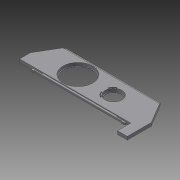
# Autodesk Inventor part: Ti Transmitted Slider
Saved by Autodesk Inventor 2013 (Build 170138000, 138)
## iProperties
Created: 2013-06-03
Part Number: Ti Transmitted Slider
Material: Generic
Document SubType Name: Modeling
Designer: kthorn
Density: 1 g/cm^3
Author: kthorn
Autodesk Inventor part; units mm, degrees
ref_plane "YZ Plane" through (0, 0, 0) normal (1, 0, 0) x (0, 1, 0)
ref_plane "XZ Plane" through (0, 0, 0) normal (0, 1, 0) x (-1, 0, 0)
ref_plane "XY Plane" through (0, 0, 0) normal (0, 0, 1) x (1, 0, 0)
sketch "Sketch1" plane through (0, 0, 0) normal (0, 0, 1) x (1, 0, 0)
  line L0 (165.1282, -41.3427) -> (-17.8718, -41.3427)
  line L1 (-17.8718, -41.3427) -> (-17.8718, -25.1427)
  line L2 (2.1282, 8.6573) -> (145.1282, 8.6573)
  line L3 (165.1282, -25.1427) -> (165.1282, -41.3427)
  line L4 (-17.8718, -25.1427) -> (2.1282, 8.6573)
  line L5 (73.6282, -41.3427) -> (73.6282, 8.6573) construction
  line L6 (165.1282, -25.1427) -> (145.1282, 8.6573)
  line L7 (165.1282, -41.3427) -> (150.3282, -41.3427)
  line L8 (150.3282, -41.3427) -> (150.3282, -61.3427)
  line L9 (150.3282, -61.3427) -> (165.1282, -61.3427)
  line L10 (165.1282, -61.3427) -> (165.1282, -41.3427)
  point P0 (0, 0)
  dimension "d2" = 16.2
  dimension "d4" = 143
  dimension "d5" = 183
  dimension "d6" = 50
  dimension "d7" = 14.8
  dimension "d8" = 20
  constraints: 22 end point, 4 parallel, 2 horizontal, 2 midpoint, 2 perpendicular, 2 symmetric about line
  measures "d2" distance of L1.end L0.end
  measures "d4" distance of L2.start L2.end
  measures "d5" distance of L0.start L0.end
  measures "d6" distance between parallel lines of L0 L2
  measures "d7" distance of L8.end L9.end
  measures "d8" distance of L7.end L8.end
extrude "Extrusion1" add sketch "Sketch1" along normal blind 5
sketch "Sketch2" plane through (0, 0, 5) normal (0, 0, 1) x (1, 0, 0)
  line L0 (165.1282, -25.1427) -> (145.1282, 8.6573) projected
  line L1 (145.1282, 8.6573) -> (2.1282, 8.6573) projected
  line L2 (2.1282, 8.6573) -> (-17.8718, -25.1427) projected
  line L3 (2.1282, 8.6573) -> (145.1282, 8.6573)
  line L4 (146.7554, 5.9073) -> (0.5009, 5.9073)
  line L5 (2.1282, 8.6573) -> (0.5009, 5.9073)
  line L6 (145.1282, 8.6573) -> (146.7554, 5.9073)
  point P0 (0, 0)
  dimension "d11" = 2.75
  constraints: 8 end point, 3 point on line, 2 collinear, 1 horizontal, 1 parallel
  measures "d11" distance between parallel lines of L4 L1
extrude "Extrusion2" cut sketch "Sketch2" against normal blind 1.2
sketch "Sketch3" plane through (0, 0, 0) normal (0, 0, -1) x (-1, 0, 0)
  line L0 (-2.1282, 8.6573) -> (17.8718, -25.1427) projected
  line L1 (-145.1282, 8.6573) -> (-2.1282, 8.6573) projected
  line L2 (-165.1282, -25.1427) -> (-145.1282, 8.6573) projected
  line L3 (-145.1282, 8.6573) -> (-2.1282, 8.6573)
  line L4 (-0.5009, 5.9073) -> (-146.7554, 5.9073)
  dimension "d17" = 2.75
  constraints: 4 end point, 2 point on line, 1 collinear, 1 parallel
  measures "d17" distance between parallel lines of L3 L4
extrude "Extrusion3" cut sketch "Sketch3" against normal blind 1.2
sketch "Sketch4" plane through (-17.8718, -41.3427, 0) normal (0, -1, 0) x (1, 0, 0)
  line L0 (163, 3.8) -> (20, 3.8)
  line L1 (20, 3.8) -> (20, 1.2)
  line L2 (20, 1.2) -> (163, 1.2)
  line L3 (163, 1.2) -> (163, 3.8)
  line L4 (163, 3.8) -> (20, 1.2) construction
  line L5 (20, 3.8) -> (163, 1.2) construction
  line L6 (168.2, 0) -> (183, 0) projected
  line L7 (183, 0) -> (183, 5) projected
  line L8 (168.2, 5) -> (183, 5) projected
  line L9 (168.2, 0) -> (168.2, 5) projected
  line L10 (168.2, 5) -> (183, 5) projected
  line L11 (0, 0) -> (183, 5) construction
  line L12 (183, 0) -> (0, 5) construction
  point P0 (17.8718, 0)
  point P1 (91.5, 2.5)
  point P2 (91.5, 2.5)
  dimension "d20" = 2.6
  dimension "d22" = 143
  constraints: 16 end point, 4 midpoint, 2 parallel, 1 horizontal, 1 perpendicular
  measures "d20" distance of L0.end L1.end
  measures "d22" distance of L0.start L0.end
extrude "Extrusion4" add sketch "Sketch4" along normal blind 3.8 contours L3 L2 L1 L0
sketch "Sketch5" plane through (2.1282, -41.3427, 3.8) normal (0, 0, 1) x (1, 0, 0)
  line L0 (0, 0) -> (143, 0) projected
  line L1 (0, 0) -> (0, -3.8) projected
  line L2 (143, -3.8) -> (0, -3.8) projected
  line L3 (143, 0) -> (143, -3.8) projected
  line L4 (5.125, -3.8) -> (137.875, -3.8)
  line L5 (137.875, -3.8) -> (137.875, -2.8)
  line L6 (137.875, -2.8) -> (5.125, -2.8)
  line L7 (5.125, -2.8) -> (5.125, -3.8)
  line L8 (5.125, -2.8) -> (0, -2.8) construction
  line L9 (137.875, -2.8) -> (143, -2.8) construction
  line L10 (143, 0) -> (128, 0)
  line L11 (128, 0) -> (128, -1.25)
  line L12 (128, -1.25) -> (143, -1.25)
  line L13 (143, -1.25) -> (143, 0)
  line L14 (71.5, 0) -> (71.5, -28.6928) construction
  line L15 (0, 0) -> (15, 0)
  line L16 (15, 0) -> (15, -1.25)
  line L17 (15, -1.25) -> (0, -1.25)
  line L18 (0, -1.25) -> (0, 0)
  line L19 (143, -2.4854) -> (140.4375, -3.8)
  line L20 (140.4375, -3.8) -> (143, -3.8)
  line L21 (143, -2.4854) -> (143, -3.8)
  line L22 (0, -2.4854) -> (2.5625, -3.8)
  line L23 (2.5625, -3.8) -> (0, -3.8)
  line L24 (0, -2.4854) -> (0, -3.8)
  point P0 (-2.1282, 41.3427)
  dimension "d25" = 1
  dimension "d27" = 132.75
  dimension "d28" = 15
  dimension "d29" = 1.25
  constraints: 42 end point, 5 parallel, 5 perpendicular, 5 point on line, 5 symmetric about line, 2 collinear, 2 horizontal, 1 midpoint
  measures "d25" distance of L6.end L4.start
  measures "d27" distance of L5.end L6.end
  measures "d28" distance of L0.end L10.end
  measures "d29" distance of L10.end L11.end
extrude "Extrusion5" cut sketch "Sketch5" against normal through all contours L0 L16 L17 L1 | L0 L3 L12 L11 | L22 L2 L1 | L7 L6 L5 L2 | L3 L2 L19
sketch "Sketch6" plane through (0, 0, 5) normal (0, 0, 1) x (1, 0, 0)
  line L0 (-17.8718, -25.1427) -> (-17.8718, -41.3427) projected
  line L1 (165.1282, -61.3427) -> (165.1282, -25.1427) projected
  line L2 (-17.8718, -41.3427) -> (165.1282, -41.3427) construction
  line L3 (165.1282, -41.3427) -> (165.1282, 5.9073) construction
  line L4 (165.1282, 5.9073) -> (-17.8718, 5.9073) construction
  line L5 (-17.8718, 5.9073) -> (-17.8718, -41.3427) construction
  line L6 (-17.8718, 5.9073) -> (165.1282, -41.3427) construction
  line L7 (-17.8718, -41.3427) -> (165.1282, 5.9073) construction
  circle A0 centre (46.6282, -17.7177) radius 22.5
  circle A1 centre (100.6282, -17.7177) radius 12.75
  line L8 (-17.8718, -17.7177) -> (165.1282, -17.7177) construction
  line L9 (46.6282, -17.7177) -> (46.6282, -36.6137) construction
  line L10 (46.6282, -36.6137) -> (-17.8718, -36.6137) construction
  line L11 (100.6282, -17.7177) -> (100.6282, -34.8345) construction
  line L12 (100.6282, -34.8345) -> (165.1282, -34.8345) construction
  circle A2 centre (46.6282, -17.7177) radius 21.5
  circle A3 centre (100.6282, -17.7177) radius 11.75
  line L13 (46.6282, 3.7823) -> (46.6282, 4.7823) construction
  line L14 (100.6282, -5.9677) -> (100.6282, -4.9677) construction
  point P0 (0, 0)
  point P1 (73.6282, -17.7177)
  dimension "d32" = 45
  dimension "d35" = 25.5
  dimension "d37" = 64.5
  dimension "d38" = 64.5
  dimension "d39" = 1
  dimension "d40" = 1
  dimension "d87" = 27
  constraints: 26 end point, 6 perpendicular, 4 point on line, 4 vertical alignment, 3 midpoint, 3 parallel, 2 coincident, 1 horizontal, 8 other
  measures "d37" distance of L9.end L10.end
  measures "d38" distance of L11.end L12.end
  measures "d39" distance of L13.start L13.end
  measures "d40" distance of L14.start L14.end
  measures "d87" distance of point (73.628, -17.718) L9.start
extrude "Extrusion6" cut sketch "Sketch6" against normal through all contours A2 | A3
extrude "Extrusion7" cut sketch "Sketch6" against normal blind 4.5
sketch "Sketch11" plane through (0, 0, 5) normal (0, 0, 1) x (1, 0, 0)
  circle A0 centre (100.6282, -17.7177) radius 12.75 projected
  line L0 (165.1282, -61.3427) -> (165.1282, -25.1427) projected
  circle A1 centre (100.6282, -17.7177) radius 13.75 construction
  circle A2 centre (100.6282, -17.7177) radius 14.75 construction
  line L1 (100.6282, -17.7177) -> (93.2532, -4.9439) construction
  line L2 (100.6282, -17.7177) -> (142.9654, -17.7177) construction
  line L3 (100.6282, -17.7177) -> (93.2532, -30.4916) construction
  line L4 (100.6282, -17.7177) -> (86.7677, -22.7625) construction
  line L5 (100.6282, -17.7177) -> (86.7677, -12.673) construction
  line L6 (93.7532, -5.8099) -> (93.2532, -4.9439)
  line L7 (87.7074, -13.015) -> (86.7677, -12.673)
  line L8 (87.7074, -22.4205) -> (86.7677, -22.7625)
  line L9 (93.7532, -29.6256) -> (93.2532, -30.4916)
  arc A3 (86.7677, -22.7625) -> (93.2532, -30.4916) centre (100.6282, -17.7177) ccw
  arc A4 (87.7074, -22.4205) -> (93.7532, -29.6256) centre (100.6282, -17.7177) ccw
  arc A5 (93.7532, -5.8099) -> (87.7074, -13.015) centre (100.6282, -17.7177) ccw
  arc A6 (93.2532, -4.9439) -> (86.7677, -12.673) centre (100.6282, -17.7177) ccw
  point P0 (0, 0)
  dimension "d88" = 1
  dimension "d89" = 1
  dimension "d90" = 120
  dimension "d93" = 120
  dimension "d94" = 40
  dimension "d95" = 40
  constraints: 18 end point, 16 point on circle, 6 centre point, 6 coincident, 4 collinear, 4 point on line, 1 perpendicular
  measures "d88" radial gap between concentric circles of A0 A1
  measures "d89" radial gap between concentric circles of A2 A1
  measures "d90" angle of L1 L2
  measures "d93" angle of L3 L2
  measures "d94" angle of L1 L5
  measures "d95" angle of L3 L4
extrude "Extrusion13" cut sketch "Sketch11" against normal through all contours A5 L7 A6 L6 | A4 L9 A3 L8
sketch "Sketch12" plane through (0, 0, 5) normal (0, 0, 1) x (1, 0, 0)
  arc A0 (93.2532, -4.9439) -> (86.7677, -12.673) centre (100.6282, -17.7177) ccw projected
  line L0 (93.2532, -4.9439) -> (93.7532, -5.8099) projected
  line L1 (93.7532, -29.6256) -> (93.2532, -30.4916) projected
  arc A1 (86.7677, -22.7625) -> (93.2532, -30.4916) centre (100.6282, -17.7177) ccw projected
  circle A2 centre (100.6282, -17.7177) radius 12.75 projected
  line L2 (100.6282, -17.7177) -> (93.2532, -4.9439) construction
  line L3 (100.6282, -17.7177) -> (93.2532, -30.4916) construction
  line L4 (100.6282, -17.7177) -> (92.3801, -5.4894) construction
  line L5 (100.6282, -17.7177) -> (92.3801, -29.9461) construction
  circle A3 centre (100.6282, -17.7177) radius 11.75 construction
  line L6 (92.3801, -5.4894) -> (94.0577, -7.9766)
  line L7 (94.7532, -7.542) -> (93.2532, -4.9439)
  line L8 (93.2532, -30.4916) -> (94.7532, -27.8935)
  line L9 (92.3801, -29.9461) -> (94.0577, -27.4589)
  arc A4 (94.0577, -27.4589) -> (94.7532, -27.8935) centre (100.6282, -17.7177) ccw
  arc A5 (92.3801, -29.9461) -> (93.2532, -30.4916) centre (100.6282, -17.7177) ccw
  arc A6 (94.7532, -7.542) -> (94.0577, -7.9766) centre (100.6282, -17.7177) ccw
  arc A7 (93.2532, -4.9439) -> (92.3801, -5.4894) centre (100.6282, -17.7177) ccw
  point P0 (0, 0)
  dimension "d100" = 4
  dimension "d101" = 4
  constraints: 16 end point, 14 point on circle, 4 centre point, 4 coincident, 4 point on line, 3 collinear
  measures "d100" angle of L2 L4
  measures "d101" angle of L5 L3
extrude "Extrusion14" cut sketch "Sketch12" against normal through all contours L0 L7 A2 L6 A0 | A2 L7 A6 L6 | L9 A4 L8 A2 | A2 L8 L1 A1 L9
sketch "Sketch13" plane through (0, 0, 5) normal (0, 0, 1) x (1, 0, 0)
  arc A0 (92.9393, -6.3185) -> (87.7074, -13.015) centre (100.6282, -17.7177) ccw projected
  arc A1 (94.2532, -28.7596) -> (94.2532, -6.6759) centre (100.6282, -17.7177) ccw projected
  line L0 (100.6282, -17.7177) -> (92.9393, -6.3185) construction
  line L1 (100.6282, -17.7177) -> (91.7898, -7.1846) construction
  line L2 (100.6282, -17.7177) -> (92.9393, -29.117) construction
  line L3 (100.6282, -17.7177) -> (91.7898, -28.2509) construction
  line L4 (100.6282, -17.7177) -> (113.3782, -17.7177) construction
  line L5 (100.6282, -17.7177) -> (113.3607, -17.0505) construction
  line L6 (100.6282, -17.7177) -> (113.3607, -18.385) construction
  line L7 (113.3607, -18.385) -> (112.3621, -18.3327)
  line L8 (113.3607, -17.0505) -> (112.3621, -17.1028)
  line L9 (93.4985, -28.288) -> (94.0577, -27.4589) construction
  arc A2 (94.0577, -7.9766) -> (94.0577, -27.4589) centre (100.6282, -17.7177) ccw construction
  line L10 (94.0577, -7.9766) -> (93.4985, -7.1475) construction
  arc A3 (93.4985, -7.1475) -> (93.4985, -28.288) centre (100.6282, -17.7177) ccw construction
  line L11 (94.7532, -27.8935) -> (94.2532, -28.7596) construction
  arc A4 (94.2532, -28.7596) -> (94.2532, -6.6759) centre (100.6282, -17.7177) ccw construction
  line L12 (94.2532, -6.6759) -> (94.7532, -7.542) construction
  arc A5 (94.7532, -27.8935) -> (94.7532, -7.542) centre (100.6282, -17.7177) ccw construction
  arc A6 (113.3607, -18.385) -> (113.3607, -17.0505) centre (100.6282, -17.7177) ccw
  arc A7 (112.3621, -18.3327) -> (112.3621, -17.1028) centre (100.6282, -17.7177) ccw
  line L13 (94.0577, -27.4589) -> (92.9393, -29.117)
  line L14 (91.7898, -28.2509) -> (93.0754, -26.7188)
  arc A8 (93.0754, -26.7188) -> (94.0577, -27.4589) centre (100.6282, -17.7177) ccw
  arc A9 (91.7898, -28.2509) -> (92.9393, -29.117) centre (100.6282, -17.7177) ccw
  arc A10 (92.9393, -6.3185) -> (91.7898, -7.1846) centre (100.6282, -17.7177) ccw
  arc A11 (94.0577, -7.9766) -> (93.0754, -8.7167) centre (100.6282, -17.7177) ccw
  line L15 (92.9393, -6.3185) -> (94.0577, -7.9766)
  line L16 (91.7898, -7.1846) -> (93.0754, -8.7167)
  point P0 (0, 0)
  dimension "d104" = 6
  dimension "d105" = 6
  dimension "d106" = 3
  dimension "d107" = 3
  constraints: 26 end point, 19 point on circle, 6 centre point, 5 coincident, 3 collinear, 1 point on line
  measures "d104" angle of L0 L1
  measures "d105" angle of L2 L3
  measures "d106" angle of L5 L4
  measures "d107" angle of L4 L6
extrude "Extrusion16" add sketch "Sketch13" against normal blind 0.5
body "Solid1"
